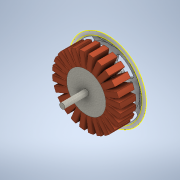
# Autodesk Inventor part: Stator3
Saved by Autodesk Inventor 2020.2 (Build 242310000, 310)
## iProperties
Created: 2020-02-19
Part Number: Stator3
Material: Copper
Document SubType Name: Modeling
Designer: user
Density: 8.94 g/cm^3
Appearance: Copper - Satin
Mass: 240.342 g
Surface Area: 187.499 cm^2
Volume: 26.8838 cm^3
Author: user
Autodesk Inventor part; units mm, degrees
ref_plane "YZ Plane" through (0, 0, 0) normal (1, 0, 0) x (0, 1, 0)
ref_plane "XZ Plane" through (0, 0, 0) normal (0, 1, 0) x (-1, 0, 0)
sketch "Sketch1" plane through (0, 0, 0) normal (1, 0, 0) x (0, 1, 0)
  line L0 (29.5, 4.8218) -> (22.5, 0)
  line L1 (22.5, 0) -> (0, 0)
  line L2 (0, 33.5) -> (0, 30)
  line L3 (27, 5.5283) -> (21.8778, 2)
  line L4 (21.8778, 2) -> (0, 2)
  line L5 (27, 5.5283) -> (29.5, 4.8218)
  line L6 (0, 0) -> (0, 2)
  point P0 (12.5, 33.5)
  point P1 (29.5, 25.3218)
  dimension "d5" = 8.5
  dimension "d9" = 2
  dimension "d10" = 2
  dimension "d11" = 22.5
  constraints: 14 end point, 3 coincident, 1 parallel, 1 vertical
  measures "d5" distance of L0.start L0.end
  measures "d9" distance between parallel lines of L0 L3
  measures "d10" distance between parallel lines of L1 L4
  measures "d11" distance of L6.start L0.end
revolve "Revolution1" add sketch "Sketch1" angle 360 about axis through (0, 0, 0) along (0, 0, 1)
sketch "Sketch2" plane through (0, 0, 0) normal (0, 0, -1) x (-1, 0, 0)
  circle A0 centre (0, 0) radius 29.5 projected
  line L0 (28.3229, -8.25) -> (28.3229, 8.25)
  line L1 (28.3229, 8.25) -> (21.5, 8.25) construction
  line L2 (21.5, 8.25) -> (21.5, 0) construction
  spline S0 degree 2 poles (28.3229, 8.25) (21.5, 8.25) (21.5, 0) knots 1 1 1 2 2 2
  line L3 (0, 0) -> (29.5, 0)
  line L4 (28.3229, -8.25) -> (21.5, -8.25) construction
  line L5 (21.5, -8.25) -> (21.5, 0) construction
  spline S1 degree 2 poles (28.3229, -8.25) (21.5, -8.25) (21.5, 0) knots 1 1 1 2 2 2
  dimension "d13" = 16.5
  dimension "d15" = 8
  constraints: 4 end point, 3 point on circle, 2 horizontal, 2 vertical, 1 symmetric about line, 6 other
  measures "d13" distance of L0.start L0.end
  measures "d15" distance of L3.end L2.end
sketch3d "3D Sketch1"
ref_plane "Work Plane1" through (-28.3229, -8.25, 4.8218) normal (0, 0, -1) x (-1, 0, 0)
extrude "Extrusion1" cut sketch "Sketch2" against normal up to surface (4.8218 mm away) contours L3 L0 A0 | A0 L0 L3 | L0 L3 S0 | S1 L3 L0
pattern_circular "Circular Pattern1" count 8 over 360 about axis through (0, 0, -10) along (0, 0, 1) of "Extrusion1"
sketch "Sketch3" plane through (-21.7173, -2.106, 0) normal (0, 0, -1) x (-1, 0, 0)
  arc A0 (0.3896, 6.2933) -> (-3.1245, 14.7771) centre (-21.7173, 2.106) ccw projected
  circle A1 centre (-21.7173, 2.106) radius 12.5
  circle A2 centre (-21.7173, 2.106) radius 16
  line L0 (-21.7173, 2.106) -> (-21.7175, 23.606)
  line L1 (-21.7173, 2.106) -> (-6.5145, 17.3088)
  point P0 (-21.7173, 23.606)
  point P1 (-25.9046, 24.2129)
  point P2 (-21.7173, 14.606)
  point P3 (-10.4036, 13.4197)
  dimension "d21" = 25
  dimension "d22" = 32
  constraints: 4 end point, 2 coincident, 1 point on line, 1 vertical alignment, 7 other
hole "Hole1" at (0, 12.5, 0) direction (0, 0, 1) diameter 2.013 end through all thread size "M2.5x0.45" class "6H" standard "ANSI Metric M Profile"
hole "Hole2" at (-11.3137, 11.3137, 0) direction (0, 0, 1) diameter 2.013 depth 7.6 tip angle 118 thread size "M2.5x0.45" class "6H" standard "ANSI Metric M Profile"
pattern_circular "Circular Pattern2" count 4 over 360 about axis through (0, 0, -10) along (0, 0, 1) of "Hole1"
pattern_circular "Circular Pattern3" count 3 over 360 about axis through (0, 0, -10) along (0, 0, 1) of "Hole2"
sketch "Sketch4" plane through (-21.7173, -2.106, 0) normal (0, 0, -1) x (-1, 0, 0)
  arc A0 (0.3896, 6.2933) -> (-3.1245, 14.7771) centre (-21.7173, 2.106) ccw projected
  arc A1 (-25.9687, 12.2512) -> (-30.8638, 8.2167) centre (-21.7173, 2.106) ccw
  arc A2 (-28.5301, 20.3771) -> (-38.3511, 12.2829) centre (-21.7173, 2.106) ccw
  line L0 (-18.6345, 14.5758) -> (-17.5449, 18.9832)
  line L1 (-24.8002, 14.5758) -> (-25.8898, 18.9832)
  line L2 (-14.3307, 12.6149) -> (-11.7199, 16.3292)
  line L3 (-11.2084, 9.4926) -> (-7.4941, 12.1034)
  arc A3 (-16.8516, 11.9713) -> (-17.4659, 12.2512) centre (-21.7173, 2.106) ccw
  arc A4 (-12.4006, 19.2363) -> (-14.9046, 20.3771) centre (-21.7173, 2.106) ccw
  line L4 (-9.2475, 5.1888) -> (-4.8401, 6.2784)
  line L5 (-9.2475, -0.9769) -> (-4.8401, -2.0665)
  line L6 (-16.3097, -9.5455) -> (-14.3983, -13.6637)
  line L7 (-24.8002, -10.3638) -> (-25.8898, -14.7713)
  line L8 (-34.1871, -0.9769) -> (-38.5945, -2.0665)
  line L9 (-33.3688, 7.5136) -> (-37.487, 9.4249)
  arc A5 (-31.8626, -2.1455) -> (-25.9687, -8.0393) centre (-21.7173, 2.106) ccw
  arc A6 (-15.6066, -7.0406) -> (-11.5721, -2.1455) centre (-21.7173, 2.106) ccw
  arc A7 (-11.5721, 6.3574) -> (-11.852, 6.9717) centre (-21.7173, 2.106) ccw
  arc A8 (-3.4461, 8.9187) -> (-4.587, 11.4227) centre (-21.7173, 2.106) ccw
  arc A9 (-11.5404, -14.5278) -> (-3.4461, -4.7068) centre (-21.7173, 2.106) ccw
  arc A10 (-39.9885, -4.7068) -> (-28.5301, -16.1652) centre (-21.7173, 2.106) ccw
  arc A11 (-25.9687, 12.2512) -> (-24.8002, 14.5758) centre (-26.7417, 14.0958) ccw
  arc A12 (-33.3688, 7.5136) -> (-30.8638, 8.2167) centre (-32.5268, 9.3278) ccw
  arc A13 (-38.3511, 12.2829) -> (-37.487, 9.4249) centre (-36.645, 11.2391) ccw
  arc A14 (-25.8898, 18.9832) -> (-28.5301, 20.3771) centre (-27.8314, 18.5032) ccw
  arc A15 (-14.9046, 20.3771) -> (-17.5449, 18.9832) centre (-15.6033, 18.5032) ccw
  arc A16 (-11.7199, 16.3292) -> (-12.4006, 19.2363) centre (-13.3561, 17.4793) ccw
  arc A17 (-16.8516, 11.9713) -> (-14.3307, 12.6149) centre (-15.9669, 13.765) ccw
  arc A18 (-18.6345, 14.5758) -> (-17.4659, 12.2512) centre (-16.6929, 14.0958) ccw
  arc A19 (-4.587, 11.4227) -> (-7.4941, 12.1034) centre (-6.344, 10.4672) ccw
  arc A20 (-4.8401, 6.2784) -> (-3.4461, 8.9187) centre (-5.3201, 8.22) ccw
  arc A21 (-11.5721, 6.3574) -> (-9.2475, 5.1888) centre (-9.7275, 7.1304) ccw
  arc A22 (-9.2475, -0.9769) -> (-11.5721, -2.1455) centre (-9.7275, -2.9184) ccw
  arc A23 (-11.2084, 9.4926) -> (-11.852, 6.9717) centre (-10.0583, 7.8564) ccw
  arc A24 (-15.6066, -7.0406) -> (-16.3097, -9.5455) centre (-14.4955, -8.7036) ccw
  arc A25 (-14.3983, -13.6637) -> (-11.5404, -14.5278) centre (-12.5842, -12.8217) ccw
  arc A26 (-3.4461, -4.7068) -> (-4.8401, -2.0665) centre (-5.3201, -4.0081) ccw
  arc A27 (-31.8626, -2.1455) -> (-34.1871, -0.9769) centre (-33.7071, -2.9184) ccw
  arc A28 (-38.5945, -2.0665) -> (-39.9885, -4.7068) centre (-38.1145, -4.0081) ccw
  arc A29 (-28.5301, -16.1652) -> (-25.8898, -14.7713) centre (-27.8314, -14.2913) ccw
  arc A30 (-24.8002, -10.3638) -> (-25.9687, -8.0393) centre (-26.7417, -9.8838) ccw
  point P0 (-17.0373, 21.036)
  point P1 (-26.3973, 21.036)
  point P2 (-19.0773, 12.7845)
  point P3 (-24.3573, 12.7845)
  point P4 (-10.5039, 18.0593)
  point P5 (-5.764, 13.3194)
  point P6 (-15.3918, 11.1053)
  point P7 (-12.718, 8.4315)
  point P8 (-2.7873, 6.786)
  point P9 (-2.7873, -2.574)
  point P10 (-13.5081, -15.5819)
  point P11 (-26.3973, -16.8241)
  point P12 (-40.6474, -2.574)
  point P13 (-39.4051, 10.3152)
  point P14 (-11.0388, 4.746)
  point P15 (-11.0388, -0.534)
  point P16 (-17.0865, -7.8718)
  point P17 (-24.3573, -8.5725)
  point P18 (-32.3958, -0.534)
  point P19 (-31.6951, 6.7368)
  dimension "d54" = 2
  constraints: 100 point on circle, 40 tangent, 30 centre point, 20 end point, 20 point on line, 19 equal radius, 2 coincident, 1 perpendicular
  measures "d54" radius of A11
extrude "Extrusion2" cut sketch "Sketch4" against normal through all
sketch3d "3D Sketch2"
sketch3d "3D Sketch3"
sketch "Sketch6" plane through (-21.7173, -2.106, 0) normal (0, 0, -1) x (-1, 0, 0)
  arc A0 (0.3896, 6.2933) -> (-3.1245, 14.7771) centre (-21.7173, 2.106) ccw projected
  circle A1 centre (-21.7173, 2.106) radius 3
  dimension "d64" = 6
  constraints: 1 centre point, 1 coincident
  measures "d64" diameter of A1
extrude "Extrusion3" add sketch "Sketch6" along normal blind 3
sketch "Sketch7" plane through (-21.5779, 1.3359, 2) normal (0, 0, 1) x (1, 0, 0)
  arc A0 (11.7125, 3.5299) -> (11.4326, 2.9155) centre (21.5779, -1.3359) ccw projected
  arc A1 (11.4326, -5.5873) -> (15.4671, -10.4824) centre (21.5779, -1.3359) ccw projected
  arc A2 (17.3264, 8.8093) -> (16.7121, 8.5294) centre (21.5779, -1.3359) ccw projected
  arc A3 (25.8293, -11.4811) -> (31.7231, -5.5873) centre (21.5779, -1.3359) ccw projected
  arc A4 (30.7244, 4.7749) -> (25.8293, 8.8093) centre (21.5779, -1.3359) ccw projected
  arc A5 (18.9108, 20.3788) -> (8.1092, 15.9046) centre (21.5779, -1.3359) ccw projected
  circle A6 centre (21.5779, -1.3359) radius 11
  point P0 (11.4326, 2.9155)
  point P1 (11.4326, -5.5873)
  point P2 (15.4671, -10.4824)
  point P3 (25.8293, -11.4811)
  point P4 (31.7231, -5.5873)
  point P5 (30.7244, 4.7749)
  point P6 (25.8293, 8.8093)
  point P7 (16.7121, 8.5294)
  point P8 (11.7125, 3.5299)
  constraints: 1 centre point, 1 coincident
extrude "Extrusion4" add sketch "Sketch7" along normal up to surface (2.8218 mm away) separate body
sketch "Sketch9" plane through (0, 0, 4.8218) normal (0, 0, 1) x (1, 0, 0)
  circle A0 centre (0, 0) radius 11 projected
extrude "Extrusion6" add sketch "Sketch9" along normal blind 16.25 bodies 2
sketch "Sketch10" plane through (0, 0, 21.0718) normal (0, 0, 1) x (1, 0, 0)
  circle A0 centre (0, 0) radius 11 projected
  circle A1 centre (0, 0) radius 3 projected
  circle A2 centre (0, 0) radius 15
  dimension "d73" = 30
  constraints: 1 centre point, 1 coincident
  measures "d73" diameter of A2
extrude "Extrusion7" add sketch "Sketch10" against normal blind 12 contours A2 bodies 2
sketch "Sketch11" plane through (0, 0, 21.0718) normal (0, 0, 1) x (1, 0, 0)
  circle A0 centre (0, 0) radius 15 projected
  circle A1 centre (0, 0) radius 26
  line L0 (15, 0) -> (26, 0)
  dimension "d76" = 52
  constraints: 2 end point, 2 horizontal alignment, 1 coincident, 1 horizontal, 3 other
extrude "Extrusion8" add sketch "Sketch11" against normal blind 12 separate body
sketch "Sketch12" plane through (0, 0, 21.0718) normal (0, 0, 1) x (1, 0, 0)
  circle A0 centre (0, 0) radius 26 projected
  circle A1 centre (0, 0) radius 15 projected
  line L0 (15, 0) -> (26, 0)
  line L1 (14.8717, 1.9579) -> (25.7776, 3.3937)
  line L2 (14.4889, 3.8823) -> (25.1141, 6.7293)
  line L3 (13.8582, 5.7403) -> (24.0209, 9.9498)
  line L4 (12.9904, 7.5) -> (22.5167, 13)
  line L5 (11.9003, 9.1314) -> (20.6272, 15.8278)
  line L6 (10.6066, 10.6066) -> (18.3848, 18.3848)
  line L7 (9.1314, 11.9003) -> (15.8278, 20.6272)
  line L8 (7.5, 12.9904) -> (13, 22.5167)
  line L9 (5.7403, 13.8582) -> (9.9498, 24.0209)
  line L10 (3.8823, 14.4889) -> (6.7293, 25.1141)
  line L11 (1.9579, 14.8717) -> (3.3937, 25.7776)
  line L12 (0, 15) -> (0, 26)
  line L13 (-1.9579, 14.8717) -> (-3.3937, 25.7776)
  line L14 (-3.8823, 14.4889) -> (-6.7293, 25.1141)
  line L15 (-5.7403, 13.8582) -> (-9.9498, 24.0209)
  line L16 (-7.5, 12.9904) -> (-13, 22.5167)
  line L17 (-9.1314, 11.9003) -> (-15.8278, 20.6272)
  line L18 (-10.6066, 10.6066) -> (-18.3848, 18.3848)
  line L19 (-11.9003, 9.1314) -> (-20.6272, 15.8278)
  line L20 (-12.9904, 7.5) -> (-22.5167, 13)
  line L21 (-13.8582, 5.7403) -> (-24.0209, 9.9498)
  line L22 (-14.4889, 3.8823) -> (-25.1141, 6.7293)
  line L23 (-14.8717, 1.9579) -> (-25.7776, 3.3937)
  line L24 (-15, 0) -> (-26, 0)
  line L25 (-14.8717, -1.9579) -> (-25.7776, -3.3937)
  line L26 (-14.4889, -3.8823) -> (-25.1141, -6.7293)
  line L27 (-13.8582, -5.7403) -> (-24.0209, -9.9498)
  line L28 (-12.9904, -7.5) -> (-22.5167, -13)
  line L29 (-11.9003, -9.1314) -> (-20.6272, -15.8278)
  line L30 (-10.6066, -10.6066) -> (-18.3848, -18.3848)
  line L31 (-9.1314, -11.9003) -> (-15.8278, -20.6272)
  line L32 (-7.5, -12.9904) -> (-13, -22.5167)
  line L33 (-5.7403, -13.8582) -> (-9.9498, -24.0209)
  line L34 (-3.8823, -14.4889) -> (-6.7293, -25.1141)
  line L35 (-1.9579, -14.8717) -> (-3.3937, -25.7776)
  line L36 (0, -15) -> (0, -26)
  line L37 (1.9579, -14.8717) -> (3.3937, -25.7776)
  line L38 (3.8823, -14.4889) -> (6.7293, -25.1141)
  line L39 (5.7403, -13.8582) -> (9.9498, -24.0209)
  line L40 (7.5, -12.9904) -> (13, -22.5167)
  line L41 (9.1314, -11.9003) -> (15.8278, -20.6272)
  line L42 (10.6066, -10.6066) -> (18.3848, -18.3848)
  line L43 (11.9003, -9.1314) -> (20.6272, -15.8278)
  line L44 (12.9904, -7.5) -> (22.5167, -13)
  line L45 (13.8582, -5.7403) -> (24.0209, -9.9498)
  line L46 (14.4889, -3.8823) -> (25.1141, -6.7293)
  line L47 (14.8717, -1.9579) -> (25.7776, -3.3937)
  line L48 (15, 0) -> (25.9599, 1.4429)
  line L49 (15, 0) -> (25.9599, -1.4429)
  dimension "d81" = 360
  constraints: 100 end point, 3 point on circle, 2 coincident, 1 horizontal, 1 horizontal alignment, 1 parallel, 193 other
extrude "Extrusion9" cut sketch "Sketch12" against normal blind 12 contours L0 L48 A0 | A0 L49 L0 bodies 3
pattern_circular "Circular Pattern4" count 24 over 360 about axis through (0, 0, -10) along (0, 0, 1) of "Extrusion9" bodies 3
sketch "Sketch13" plane through (0, 0, 21.0718) normal (0, 0, 1) x (1, 0, 0)
  circle A0 centre (0, 0) radius 15 projected
  circle A1 centre (0, 0) radius 2
  dimension "d88" = 4
  constraints: 1 centre point, 1 coincident
  measures "d88" diameter of A1
extrude "Extrusion10" add sketch "Sketch13" along normal blind 4.25 contours A1 bodies 2
sketch "Sketch14" plane through (0, 0, 25.3218) normal (0, 0, 1) x (1, 0, 0)
  circle A0 centre (0, 0) radius 2 projected
extrude "Extrusion11" add sketch "Sketch14" along normal blind 14.178 bodies 2
equation "\"d10\" = d9"
body "Solid1"
body "Solid2"
body "Solid3"
